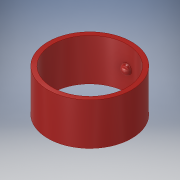
# Autodesk Inventor part: ExternalMotorizedOuterRing
Saved by Autodesk Inventor 2019.3 (Build 233278000, 278)
## iProperties
Created: 2018-12-30
Part Number: ExternalMotorizedOuterRing
Material: PET Plastic
Document SubType Name: Modeling
Designer: steele
Density: 1.541 g/cm^3
Appearance: Orange-Red
Author: steele
Autodesk Inventor part; units mm, degrees
ref_plane "YZ Plane" through (0, 0, 0) normal (1, 0, 0) x (0, 1, 0)
ref_plane "XZ Plane" through (0, 0, 0) normal (0, 1, 0) x (-1, 0, 0)
ref_plane "XY Plane" through (0, 0, 0) normal (0, 0, 1) x (1, 0, 0)
sketch "Sketch1" plane through (0, 0, 0) normal (0, 1, 0) x (-1, 0, 0)
  circle A0 centre (0, 0) radius 22.606
  circle A1 centre (0, 0) radius 25.273
  dimension "d0" = 45.212
  dimension "d1" = 50.546
  constraints: 2 centre point, 2 coincident
  measures "d0" diameter of A0
  measures "d1" diameter of A1
extrude "Extrusion1" add sketch "Sketch1" along normal mid plane 25.4
sketch "Sketch5" plane through (0, 0, 0) normal (1, 0, 0) x (0, 1, 0)
  line L0 (-12.7, -22.606) -> (12.7, -22.606) projected
  arc A0 (0, -25.527) -> (0, -19.685) centre (0, -22.606) ccw
  line L1 (0, -25.527) -> (0, -19.685)
  line L2 (0, -25.527) -> (0, -19.685) construction
  point P0 (0, 0)
  dimension "d7" = 2.921
  constraints: 4 end point, 3 point on circle, 1 centre point, 1 midpoint, 1 perpendicular
  measures "d7" radius of A0
revolve "Revolution2" add sketch "Sketch5" angle 360 about axis through (0, 0, -25.527) along (0, 0, 1)
body "Solid1"
